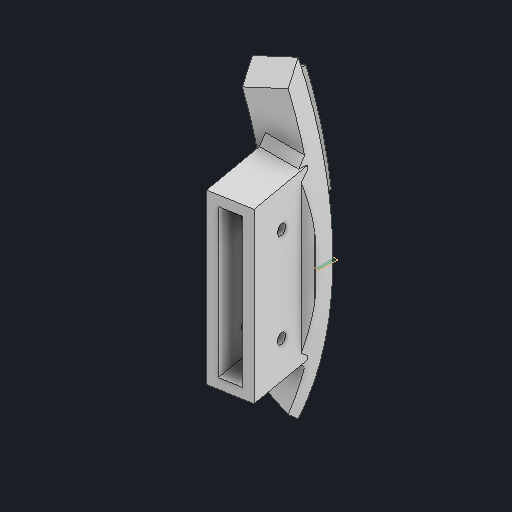
# Autodesk Inventor part: Lazercut_base
Saved by Autodesk Inventor 2023.4 (Build 274418000, 418)
## iProperties
Created: 2025-10-08
Part Number: Lazercut_base
Material: Generic
Document SubType Name: Modeling
Designer: Malthe Sennels
Density: 1 g/cm^3
Appearance: Default
Author: Malthe Sennels
Autodesk Inventor part; units mm, degrees
(part 1 of 2)
ref_plane "YZ Plane" through (0, 0, 0) normal (1, 0, 0) x (0, 1, 0)
ref_plane "XZ Plane" through (0, 0, 0) normal (0, 1, 0) x (-1, 0, 0)
ref_plane "XY Plane" through (0, 0, 0) normal (0, 0, 1) x (1, 0, 0)
sketch "Sketch1" plane through (0, 0, 0) normal (0, 0, 1) x (1, 0, 0)
  arc A0 (68.185975, 86.31728) -> (-68.185975, 86.31728) centre (0, 0) ccw
  arc A1 (5.434085, -92.914821) -> (6.399024, -89.470049) centre (-14.90414, -85.360206) ccw
  arc A2 (4.227461, -92.977534) -> (5.434085, -92.914821) centre (0, 0) ccw
  arc A3 (2.910609, -89.651355) -> (4.227461, -92.977534) centre (23.672934, -83.355206) ccw
  arc A4 (1.746562, -89.681585) -> (2.910609, -89.651355) centre (0, 0) ccw
  arc A5 (0.604127, -93.07163) -> (1.746562, -89.681585) centre (-19.314571, -84.471566) ccw
  arc A6 (-0.604127, -93.07163) -> (0.604127, -93.07163) centre (0, 0) ccw
  arc A7 (-1.746562, -89.681585) -> (-0.604127, -93.07163) centre (19.314571, -84.471566) ccw
  arc A8 (-2.910609, -89.651355) -> (-1.746562, -89.681585) centre (0, 0) ccw
  arc A9 (-4.227461, -92.977534) -> (-2.910609, -89.651355) centre (-23.672934, -83.355206) ccw
  arc A10 (-5.434085, -92.914821) -> (-4.227461, -92.977534) centre (0, 0) ccw
  arc A11 (-6.399024, -89.470049) -> (-5.434085, -92.914821) centre (14.90414, -85.360206) ccw
  arc A12 (-7.559934, -89.379442) -> (-6.399024, -89.470049) centre (0, 0) ccw
  arc A13 (-9.047651, -92.632787) -> (-7.559934, -89.379442) centre (-27.967478, -82.014135) ccw
  arc A14 (-10.249395, -92.50753) -> (-9.047651, -92.632787) centre (0, 0) ccw
  arc A15 (-11.034236, -89.017317) -> (-10.249395, -92.50753) centre (10.45353, -86.01873) ccw
  arc A16 (-12.188878, -88.866577) -> (-11.034236, -89.017317) centre (0, 0) ccw
  arc A17 (-13.843451, -92.038319) -> (-12.188878, -88.866577) centre (-32.186627, -80.451968) ccw
  arc A18 (-15.037073, -91.850856) -> (-13.843451, -92.038319) centre (0, 0) ccw
  arc A19 (-15.639701, -88.324611) -> (-15.037073, -91.850856) centre (5.974739, -86.445362) ccw
  arc A20 (-16.784963, -88.114143) -> (-15.639701, -88.324611) centre (0, 0) ccw
  arc A21 (-18.601932, -91.195731) -> (-16.784963, -88.114143) centre (-36.319007, -78.672917) ccw
  arc A22 (-19.784215, -90.946567) -> (-18.601932, -91.195731) centre (0, 0) ccw
  arc A23 (-20.203005, -87.393797) -> (-19.784215, -90.946567) centre (1.479841, -86.638954) ccw
  arc A24 (-21.335799, -87.124169) -> (-20.203005, -87.393797) centre (0, 0) ccw
  arc A25 (-23.310265, -90.107296) -> (-21.335799, -87.124169) centre (-40.353477, -76.681778) ccw
  arc A26 (-24.478021, -89.797103) -> (-23.310265, -90.107296) centre (0, 0) ccw
  arc A27 (-24.711845, -86.227385) -> (-24.478021, -89.797103) centre (-3.019046, -86.598981) ccw
  arc A28 (-25.829117, -85.899324) -> (-24.711845, -86.227385) centre (0, 0) ccw
  arc A29 (-27.955757, -88.775948) -> (-25.829117, -85.899324) centre (-44.279161, -74.483918) ccw
  arc A30 (-29.10584, -88.405562) -> (-27.955757, -88.775948) centre (0, 0) ccw
  arc A31 (-29.154066, -84.828519) -> (-29.10584, -88.405562) centre (-7.509794, -86.325554) ccw
  arc A32 (-30.252804, -84.44291) -> (-29.154066, -84.828519) centre (0, 0) ccw
  arc A33 (-32.525886, -87.205275) -> (-30.252804, -84.44291) centre (-48.085476, -72.085263) ccw
  arc A34 (-33.655194, -86.775695) -> (-32.525886, -87.205275) centre (0, 0) ccw
  arc A35 (-33.517693, -83.20097) -> (-33.655194, -86.775695) centre (-11.980297, -85.819407) ccw
  arc A36 (-34.594936, -82.758852) -> (-33.517693, -83.20097) centre (0, 0) ccw
  arc A37 (-37.008331, -85.399512) -> (-34.594936, -82.758852) centre (-51.762162, -69.492279) ccw
  arc A38 (-38.11382, -84.911896) -> (-37.008331, -85.399512) centre (0, 0) ccw
  arc A39 (-37.790962, -81.349126) -> (-38.11382, -84.911896) centre (-16.418504, -85.081907) ccw
  arc A40 (-38.843805, -80.851691) -> (-37.790962, -81.349126) centre (0, 0) ccw
  arc A41 (-41.391008, -83.363528) -> (-38.843805, -80.851691) centre (-55.299306, -66.711955) ccw
  arc A42 (-42.469697, -82.819189) -> (-41.391008, -83.363528) centre (0, 0) ccw
  arc A43 (-41.962354, -79.27798) -> (-42.469697, -82.819189) centre (-20.812449, -84.115041) ccw
  arc A44 (-42.987959, -78.726568) -> (-41.962354, -79.27798) centre (0, 0) ccw
  arc A45 (-45.662101, -81.10281) -> (-42.987959, -78.726568) centre (-58.687372, -63.751788) ccw
  arc A46 (-46.711084, -80.503217) -> (-45.662101, -81.10281) centre (0, 0) ccw
  arc A47 (-46.020622, -76.993114) -> (-46.711084, -80.503217) centre (-25.150288, -82.921416) ccw
  arc A48 (-47.016224, -76.389213) -> (-46.020622, -76.993114) centre (0, 0) ccw
  arc A49 (-49.810099, -78.623453) -> (-47.016224, -76.389213) centre (-61.917228, -60.619758) ccw
  arc A50 (-50.826546, -77.970222) -> (-49.810099, -78.623453) centre (0, 0) ccw
  arc A51 (-49.954827, -74.500688) -> (-50.826546, -77.970222) centre (-29.420325, -81.504249) ccw
  arc A52 (-50.917742, -73.845925) -> (-49.954827, -74.500688) centre (0, 0) ccw
  arc A53 (-53.823816, -75.932141) -> (-50.917742, -73.845925) centre (-64.980166, -57.324307) ccw
  arc A54 (-54.804988, -75.227033) -> (-53.823816, -75.932141) centre (0, 0) ccw
  arc A55 (-53.754362, -71.807421) -> (-54.804988, -75.227033) centre (-33.611051, -79.867362) ccw
  arc A56 (-54.681995, -71.103562) -> (-53.754362, -71.807421) centre (0, 0) ccw
  arc A57 (-57.692435, -73.03613) -> (-54.681995, -71.103562) centre (-67.867929, -53.874321) ccw
  arc A58 (-58.635686, -72.281046) -> (-57.692435, -73.03613) centre (0, 0) ccw
  arc A59 (-57.408985, -68.920574) -> (-58.635686, -72.281046) centre (-37.711167, -78.015166) ccw
  arc A60 (-58.298835, -68.169517) -> (-57.408985, -68.920574) centre (0, 0) ccw
  arc A61 (-61.405524, -69.943226) -> (-58.298835, -68.169517) centre (-70.572732, -50.279098) ccw
  arc A62 (-62.308313, -69.140201) -> (-61.405524, -69.943226) centre (0, 0) ccw
  arc A63 (-60.908844, -65.84793) -> (-62.308313, -69.140201) centre (-41.709621, -75.952654) ccw
  arc A64 (-61.758512, -65.051698) -> (-60.908844, -65.84793) centre (0, 0) ccw
  arc A65 (-64.953076, -66.661768) -> (-61.758512, -65.051698) centre (-73.087283, -46.548332) ccw
  arc A66 (-65.812967, -65.812967) -> (-64.953076, -66.661768) centre (0, 0) ccw
  arc A67 (-64.244503, -62.597771) -> (-65.812967, -65.812967) centre (-45.595633, -73.685388) ccw
  arc A68 (-65.051698, -61.758512) -> (-64.244503, -62.597771) centre (0, 0) ccw
  arc A69 (-68.325525, -63.200601) -> (-65.051698, -61.758512) centre (-75.404804, -42.69208) ccw
  arc A70 (-69.140201, -62.308313) -> (-68.325525, -63.200601) centre (0, 0) ccw
  arc A71 (-67.406971, -59.17886) -> (-69.140201, -62.308313) centre (-49.358727, -71.21948) ccw
  arc A72 (-68.169517, -58.298835) -> (-67.406971, -59.17886) centre (0, 0) ccw
  arc A73 (-71.513781, -59.569056) -> (-68.169517, -58.298835) centre (-77.519047, -38.720738) ccw
  arc A74 (-72.281046, -58.635686) -> (-71.513781, -59.569056) centre (0, 0) ccw
  arc A75 (-70.387721, -55.600413) -> (-72.281046, -58.635686) centre (-52.988759, -68.561576) ccw
  arc A76 (-71.103562, -54.681995) -> (-70.387721, -55.600413) centre (0, 0) ccw
  arc A77 (-74.509248, -55.776924) -> (-71.103562, -54.681995) centre (-79.424312, -34.645011) ccw
  arc A78 (-75.227033, -54.804988) -> (-74.509248, -55.776924) centre (0, 0) ccw
  arc A79 (-73.178718, -51.872077) -> (-75.227033, -54.804988) centre (-56.475942, -65.718842) ccw
  arc A80 (-73.845925, -50.917742) -> (-73.178718, -51.872077) centre (0, 0) ccw
  arc A81 (-77.303851, -51.834427) -> (-73.845925, -50.917742) centre (-81.115464, -30.475887) ccw
  arc A82 (-77.970222, -50.826546) -> (-77.303851, -51.834427) centre (0, 0) ccw
  arc A83 (-75.772439, -48.003903) -> (-77.970222, -50.826546) centre (-59.810876, -62.698942) ccw
  arc A84 (-76.389213, -47.016224) -> (-75.772439, -48.003903) centre (0, 0) ccw
  arc A85 (-79.890057, -47.752194) -> (-76.389213, -47.016224) centre (-82.587942, -26.224606) ccw
  arc A86 (-80.503217, -46.711084) -> (-79.890057, -47.752194) centre (0, 0) ccw
  arc A87 (-78.16189, -44.006319) -> (-80.503217, -46.711084) centre (-62.984571, -59.510016) ccw
  arc A88 (-78.726568, -42.987959) -> (-78.16189, -44.006319) centre (0, 0) ccw
  arc A89 (-82.260894, -43.541229) -> (-78.726568, -42.987959) centre (-83.837778, -21.902628) ccw
  arc A90 (-82.819189, -42.469697) -> (-82.260894, -43.541229) centre (0, 0) ccw
  arc A91 (-80.340631, -39.890102) -> (-82.819189, -42.469697) centre (-65.98847, -56.160662) ccw
  arc A92 (-80.851691, -38.843805) -> (-80.340631, -39.890102) centre (0, 0) ccw
  arc A93 (-84.409969, -39.212885) -> (-80.851691, -38.843805) centre (-84.861602, -17.521605) ccw
  arc A94 (-84.911896, -38.11382) -> (-84.409969, -39.212885) centre (0, 0) ccw
  arc A95 (-82.302787, -35.666348) -> (-84.911896, -38.11382) centre (-68.814477, -52.659909) ccw
  arc A96 (-82.758852, -34.594936) -> (-82.302787, -35.666348) centre (0, 0) ccw
  arc A97 (-86.331491, -34.77883) -> (-82.758852, -34.594936) centre (-85.656655, -13.093346) ccw
  arc A98 (-86.775695, -33.655194) -> (-86.331491, -34.77883) centre (0, 0) ccw
  arc A99 (-84.04307, -31.346444) -> (-86.775695, -33.655194) centre (-71.454971, -49.017194) ccw
  arc A100 (-84.44291, -30.252804) -> (-84.04307, -31.346444) centre (0, 0) ccw
  arc A101 (-88.020277, -30.251017) -> (-84.44291, -30.252804) centre (-86.220792, -8.62979) ccw
  arc A102 (-88.405562, -29.10584) -> (-88.020277, -30.251017) centre (0, 0) ccw
  arc A103 (-85.556787, -26.942036) -> (-88.405562, -29.10584) centre (-73.902836, -45.242337) ccw
  arc A104 (-85.899324, -25.829117) -> (-85.556787, -26.942036) centre (0, 0) ccw
  arc A105 (-89.471777, -25.641653) -> (-85.899324, -25.829117) centre (-86.552493, -4.142969) ccw
  arc A106 (-89.797103, -24.478021) -> (-89.471777, -25.641653) centre (0, 0) ccw
  arc A107 (-86.839859, -22.464997) -> (-89.797103, -24.478021) centre (-76.151471, -41.345515) ccw
  arc A108 (-87.124169, -21.335799) -> (-86.839859, -22.464997) centre (0, 0) ccw
  arc A109 (-90.682077, -20.963164) -> (-87.124169, -21.335799) centre (-86.650864, 0.35502) ccw
  arc A110 (-90.946567, -19.784215) -> (-90.682077, -20.963164) centre (0, 0) ccw
  arc A111 (-87.888826, -17.927395) -> (-90.946567, -19.784215) centre (-78.194816, -37.337233) ccw
  arc A112 (-88.114143, -16.784963) -> (-87.888826, -17.927395) centre (0, 0) ccw
  arc A113 (-91.647914, -16.228161) -> (-88.114143, -16.784963) centre (-86.515639, 4.852052) ccw
  arc A114 (-91.850856, -15.037073) -> (-91.647914, -16.228161) centre (0, 0) ccw
  arc A115 (-88.700859, -13.341465) -> (-91.850856, -15.037073) centre (-80.027361, -33.228296) ccw
  arc A116 (-88.866577, -12.188878) -> (-88.700859, -13.341465) centre (0, 0) ccw
  arc A117 (-92.366684, -11.44941) -> (-88.866577, -12.188878) centre (-86.147184, 9.336004) ccw
  arc A118 (-92.50753, -10.249395) -> (-92.366684, -11.44941) centre (0, 0) ccw
  arc A119 (-89.273772, -8.719569) -> (-92.50753, -10.249395) centre (-81.644167, -29.029782) ccw
  arc A120 (-89.379442, -7.559934) -> (-89.273772, -8.719569) centre (0, 0) ccw
  arc A121 (-92.83645, -6.639794) -> (-89.379442, -7.559934) centre (-85.546491, 13.794787) ccw
  arc A122 (-92.914821, -5.434085) -> (-92.83645, -6.639794) centre (0, 0) ccw
  arc A123 (-89.606017, -4.074166) -> (-92.914821, -5.434085) centre (-83.040874, -24.753008) ccw
  arc A124 (-89.651355, -2.910609) -> (-89.606017, -4.074166) centre (0, 0) ccw
  arc A125 (-93.055945, -1.812278) -> (-89.651355, -2.910609) centre (-84.715179, 18.216383) ccw
  arc A126 (-93.07163, -0.604127) -> (-93.055945, -1.812278) centre (0, 0) ccw
  arc A127 (-89.696701, 0.58222) -> (-93.07163, -0.604127) centre (-84.213718, -20.409505) ccw
  arc A128 (-89.681585, 1.746562) -> (-89.696701, 0.58222) centre (0, 0) ccw
  arc A129 (-93.024578, 3.020124) -> (-89.681585, 1.746562) centre (-83.655491, 22.58887) ccw
  arc A130 (-92.977534, 4.227461) -> (-93.024578, 3.020124) centre (0, 0) ccw
  arc A131 (-89.545578, 5.237036) -> (-92.977534, 4.227461) centre (-85.159537, -16.010981) ccw
  arc A132 (-89.470049, 6.399024) -> (-89.545578, 5.237036) centre (0, 0) ccw
  arc A133 (-92.742433, 7.844384) -> (-89.470049, 6.399024) centre (-82.370282, 26.900461) ccw
  arc A134 (-92.632787, 9.047651) -> (-92.742433, 7.844384) centre (0, 0) ccw
  arc A135 (-89.153057, 9.877735) -> (-92.632787, 9.047651) centre (-85.87578, -11.569295) ccw
  arc A136 (-89.017317, 11.034236) -> (-89.153057, 9.877735) centre (0, 0) ccw
  arc A137 (-92.210271, 12.647497) -> (-89.017317, 11.034236) centre (-80.863018, 31.139534) ccw
  arc A138 (-92.038319, 13.843451) -> (-92.210271, 12.647497) centre (0, 0) ccw
  arc A139 (-88.520194, 14.491805) -> (-92.038319, 13.843451) centre (-86.360518, -7.09642) ccw
  arc A140 (-88.324611, 15.639701) -> (-88.520194, 14.491805) centre (0, 0) ccw
  arc A141 (-91.429527, 17.416514) -> (-88.324611, 15.639701) centre (-79.137761, 35.29466) ccw
  arc A142 (-91.195731, 18.601932) -> (-91.429527, 17.416514) centre (0, 0) ccw
  arc A143 (-87.648697, 19.066807) -> (-91.195731, 18.601932) centre (-86.612443, -2.604414) ccw
  arc A144 (-87.393797, 20.203005) -> (-87.648697, 19.066807) centre (0, 0) ccw
  arc A145 (-90.402304, 22.13858) -> (-87.393797, 20.203005) centre (-77.199162, 39.354638) ccw
  arc A146 (-90.107296, 23.310265) -> (-90.402304, 22.13858) centre (0, 0) ccw
  arc A147 (-86.540914, 23.590409) -> (-90.107296, 23.310265) centre (-86.630876, 1.894613) ccw
  arc A148 (-86.227385, 24.711845) -> (-86.540914, 23.590409) centre (0, 0) ccw
  arc A149 (-89.131373, 26.800963) -> (-86.227385, 24.711845) centre (-75.052449, 43.308523) ccw
  arc A150 (-88.775948, 27.955757) -> (-89.131373, 26.800963) centre (0, 0) ccw
  arc A151 (-85.199832, 28.050415) -> (-88.775948, 27.955757) centre (-86.415767, 6.388533) ccw
  arc A152 (-84.828519, 29.154066) -> (-85.199832, 28.050415) centre (0, 0) ccw
  arc A153 (-87.620159, 31.391097) -> (-84.828519, 29.154066) centre (-72.703407, 47.145655) ccw
  arc A154 (-87.205275, 32.525886) -> (-87.620159, 31.391097) centre (0, 0) ccw
  arc A155 (-83.629067, 32.434802) -> (-87.205275, 32.525886) centre (-85.967697, 10.86523) ccw
  arc A156 (-83.20097, 33.517693) -> (-83.629067, 32.434802) centre (0, 0) ccw
  arc A157 (-85.872737, 35.896605) -> (-83.20097, 33.517693) centre (-70.15837, 50.855692) ccw
  arc A158 (-85.399512, 37.008331) -> (-85.872737, 35.896605) centre (0, 0) ccw
  arc A159 (-81.832852, 36.73175) -> (-85.399512, 37.008331) centre (-85.287874, 15.312636) ccw
  arc A160 (-81.349126, 37.790962) -> (-81.832852, 36.73175) centre (0, 0) ccw
  arc A161 (-83.893818, 40.305343) -> (-81.349126, 37.790962) centre (-67.424198, 54.42863) ccw
  arc A162 (-83.363528, 41.391008) -> (-83.893818, 40.305343) centre (0, 0) ccw
  arc A163 (-79.816031, 40.929677) -> (-83.363528, 41.391008) centre (-84.378129, 19.718762) ccw
  arc A164 (-79.27798, 41.962354) -> (-79.816031, 40.929677) centre (0, 0) ccw
  arc A165 (-81.688735, 44.605424) -> (-79.27798, 41.962354) centre (-64.508262, 57.854838) ccw
  arc A166 (-81.10281, 45.662101) -> (-81.688735, 44.605424) centre (0, 0) ccw
  arc A167 (-77.584039, 45.017264) -> (-81.10281, 45.662101) centre (-83.240915, 24.07173) ccw
  arc A168 (-76.993114, 46.020622) -> (-77.584039, 45.017264) centre (0, 0) ccw
  arc A169 (-79.263434, 48.785257) -> (-76.993114, 46.020622) centre (-61.418424, 61.12508) ccw
  arc A170 (-78.623453, 49.810099) -> (-79.263434, 48.785257) centre (0, 0) ccw
  arc A171 (-75.142895, 48.983492) -> (-78.623453, 49.810099) centre (-81.879299, 28.359805) ccw
  arc A172 (-74.500688, 49.954827) -> (-75.142895, 48.983492) centre (0, 0) ccw
  arc A173 (-76.624453, 52.833574) -> (-74.500688, 49.954827) centre (-58.163012, 64.23054) ccw
  arc A174 (-75.932141, 53.823816) -> (-76.624453, 52.833574) centre (0, 0) ccw
  arc A175 (-72.499179, 52.81767) -> (-75.932141, 53.823816) centre (-80.296951, 32.571427) ccw
  arc A176 (-71.807421, 53.754362) -> (-72.499179, 52.81767) centre (0, 0) ccw
  arc A177 (-73.778906, 56.73946) -> (-71.807421, 53.754362) centre (-54.750803, 67.162845) ccw
  arc A178 (-73.03613, 57.692435) -> (-73.778906, 56.73946) centre (0, 0) ccw
  arc A179 (-69.660017, 56.509461) -> (-73.03613, 57.692435) centre (-78.498136, 36.695242) ccw
  arc A180 (-68.920574, 57.408985) -> (-69.660017, 56.509461) centre (0, 0) ccw
  arc A181 (-70.734464, 60.492388) -> (-68.920574, 57.408985) centre (-51.190996, 69.914091) ccw
  arc A182 (-69.943226, 61.405524) -> (-70.734464, 60.492388) centre (0, 0) ccw
  arc A183 (-66.633065, 60.048912) -> (-69.943226, 61.405524) centre (-76.487705, 40.720133) ccw
  arc A184 (-65.84793, 60.908844) -> (-66.633065, 60.048912) centre (0, 0) ccw
  arc A185 (-67.499334, 64.082238) -> (-65.84793, 60.908844) centre (-47.493187, 72.476861) ccw
  arc A186 (-66.661768, 64.953076) -> (-67.499334, 64.082238) centre (0, 0) ccw
  arc A187 (-63.426482, 63.426482) -> (-66.661768, 64.953076) centre (-74.271076, 44.63525) ccw
  arc A188 (-62.597771, 64.244503) -> (-63.426482, 63.426482) centre (0, 0) ccw
  arc A189 (-64.082238, 67.499334) -> (-62.597771, 64.244503) centre (-43.667344, 74.844247) ccw
  arc A190 (-63.200601, 68.325525) -> (-64.082238, 67.499334) centre (0, 0) ccw
  arc A191 (-60.048912, 66.633065) -> (-63.200601, 68.325525) centre (-71.854225, 48.430038) ccw
  arc A192 (-59.17886, 67.406971) -> (-60.048912, 66.633065) centre (0, 0) ccw
  arc A193 (-60.492388, 70.734464) -> (-59.17886, 67.406971) centre (-39.723782, 77.009865) ccw
  arc A194 (-59.569056, 71.513781) -> (-60.492388, 70.734464) centre (0, 0) ccw
  arc A195 (-56.509461, 69.660017) -> (-59.569056, 71.513781) centre (-69.243668, 52.094267) ccw
  arc A196 (-55.600413, 70.387721) -> (-56.509461, 69.660017) centre (0, 0) ccw
  arc A197 (-56.73946, 73.778906) -> (-55.600413, 70.387721) centre (-35.673132, 78.967878) ccw
  arc A198 (-55.776924, 74.509248) -> (-56.73946, 73.778906) centre (0, 0) ccw
  arc A199 (-52.81767, 72.499179) -> (-55.776924, 74.509248) centre (-66.446442, 55.618059) ccw
  arc A200 (-51.872077, 73.178718) -> (-52.81767, 72.499179) centre (0, 0) ccw
  arc A201 (-52.833574, 76.624453) -> (-51.872077, 73.178718) centre (-31.526314, 80.713009) ccw
  arc A202 (-51.834427, 77.303851) -> (-52.833574, 76.624453) centre (0, 0) ccw
  arc A203 (-48.983492, 75.142895) -> (-51.834427, 77.303851) centre (-63.470089, 58.991915) ccw
  arc A204 (-48.003903, 75.772439) -> (-48.983492, 75.142895) centre (0, 0) ccw
  arc A205 (-48.785257, 79.263434) -> (-48.003903, 75.772439) centre (-27.294506, 82.240551) ccw
  arc A206 (-47.752194, 79.890057) -> (-48.785257, 79.263434) centre (0, 0) ccw
  arc A207 (-45.017264, 77.584039) -> (-47.752194, 79.890057) centre (-60.322631, 62.206739) ccw
  arc A208 (-44.006319, 78.16189) -> (-45.017264, 77.584039) centre (0, 0) ccw
  arc A209 (-44.605424, 81.688735) -> (-44.006319, 78.16189) centre (-22.989116, 83.546387) ccw
  arc A210 (-43.541229, 82.260894) -> (-44.605424, 81.688735) centre (0, 0) ccw
  arc A211 (-40.929677, 79.816031) -> (-43.541229, 82.260894) centre (-57.012554, 65.253865) ccw
  arc A212 (-39.890102, 80.340631) -> (-40.929677, 79.816031) centre (0, 0) ccw
  arc A213 (-40.305343, 83.893818) -> (-39.890102, 80.340631) centre (-18.621753, 84.626996) ccw
  arc A214 (-39.212885, 84.409969) -> (-40.305343, 83.893818) centre (0, 0) ccw
  arc A215 (-36.73175, 81.832852) -> (-39.212885, 84.409969) centre (-53.548782, 68.125078) ccw
  arc A216 (-35.666348, 82.302787) -> (-36.73175, 81.832852) centre (0, 0) ccw
  arc A217 (-35.896605, 85.872737) -> (-35.666348, 82.302787) centre (-14.204188, 85.479467) ccw
  arc A218 (-34.77883, 86.331491) -> (-35.896605, 85.872737) centre (0, 0) ccw
  arc A219 (-32.434802, 83.629067) -> (-34.77883, 86.331491) centre (-49.940651, 70.812637) ccw
  arc A220 (-31.346444, 84.04307) -> (-32.434802, 83.629067) centre (0, 0) ccw
  arc A221 (-31.391097, 87.620159) -> (-31.346444, 84.04307) centre (-9.748331, 86.1015) ccw
  arc A222 (-30.251017, 88.020277) -> (-31.391097, 87.620159) centre (0, 0) ccw
  arc A223 (-28.050415, 85.199832) -> (-30.251017, 88.020277) centre (-46.197889, 73.309298) ccw
  arc A224 (-26.942036, 85.556787) -> (-28.050415, 85.199832) centre (0, 0) ccw
  arc A225 (-26.800963, 89.131373) -> (-26.942036, 85.556787) centre (-5.266195, 86.491418) ccw
  arc A226 (-25.641653, 89.471777) -> (-26.800963, 89.131373) centre (0, 0) ccw
  arc A227 (-23.590409, 86.540914) -> (-25.641653, 89.471777) centre (-42.330586, 75.608331) ccw
  arc A228 (-22.464997, 86.839859) -> (-23.590409, 86.540914) centre (0, 0) ccw
  arc A229 (-22.13858, 90.402304) -> (-22.464997, 86.839859) centre (-0.769862, 86.648171) ccw
  arc A230 (-20.963164, 90.682077) -> (-22.13858, 90.402304) centre (0, 0) ccw
  arc A231 (-19.066807, 87.648697) -> (-20.963164, 90.682077) centre (-38.349167, 77.703537) ccw
  arc A232 (-17.927395, 87.888826) -> (-19.066807, 87.648697) centre (0, 0) ccw
  arc A233 (-17.416514, 91.429527) -> (-17.927395, 87.888826) centre (3.728547, 86.571336) ccw
  arc A234 (-16.228161, 91.647914) -> (-17.416514, 91.429527) centre (0, 0) ccw
  arc A235 (-14.491805, 88.520194) -> (-16.228161, 91.647914) centre (-34.264365, 79.589267) ccw
  arc A236 (-13.341465, 88.700859) -> (-14.491805, 88.520194) centre (0, 0) ccw
  arc A237 (-12.647497, 92.210271) -> (-13.341465, 88.700859) centre (8.216904, 86.261119) ccw
  arc A238 (-11.44941, 92.366684) -> (-12.647497, 92.210271) centre (0, 0) ccw
  arc A239 (-9.877735, 89.153057) -> (-11.44941, 92.366684) centre (-30.087193, 81.260439) ccw
  arc A240 (-8.719569, 89.273772) -> (-9.877735, 89.153057) centre (0, 0) ccw
  arc A241 (-7.844384, 92.742433) -> (-8.719569, 89.273772) centre (12.68311, 85.718358) ccw
  arc A242 (-6.639794, 92.83645) -> (-7.844384, 92.742433) centre (0, 0) ccw
  arc A243 (-5.237036, 89.545578) -> (-6.639794, 92.83645) centre (-25.828911, 82.712548) ccw
  arc A244 (-4.074166, 89.606017) -> (-5.237036, 89.545578) centre (0, 0) ccw
  arc A245 (-3.020124, 93.024578) -> (-4.074166, 89.606017) centre (17.115124, 84.944516) ccw
  arc A246 (-1.812278, 93.055945) -> (-3.020124, 93.024578) centre (0, 0) ccw
  arc A247 (-0.58222, 89.696701) -> (-1.812278, 93.055945) centre (-21.500999, 83.941678) ccw
  arc A248 (0.58222, 89.696701) -> (-0.58222, 89.696701) centre (0, 0) ccw
  arc A249 (1.812278, 93.055945) -> (0.58222, 89.696701) centre (21.500999, 83.941678) ccw
  arc A250 (3.020124, 93.024578) -> (1.812278, 93.055945) centre (0, 0) ccw
  arc A251 (4.074166, 89.606017) -> (3.020124, 93.024578) centre (-17.115124, 84.944516) ccw
  arc A252 (5.237036, 89.545578) -> (4.074166, 89.606017) centre (0, 0) ccw
  arc A253 (6.639794, 92.83645) -> (5.237036, 89.545578) centre (25.828911, 82.712548) ccw
  arc A254 (7.844384, 92.742433) -> (6.639794, 92.83645) centre (0, 0) ccw
  arc A255 (8.719569, 89.273772) -> (7.844384, 92.742433) centre (-12.68311, 85.718358) ccw
  arc A256 (9.877735, 89.153057) -> (8.719569, 89.273772) centre (0, 0) ccw
  arc A257 (11.44941, 92.366684) -> (9.877735, 89.153057) centre (30.087193, 81.260439) ccw
  arc A258 (12.647497, 92.210271) -> (11.44941, 92.366684) centre (0, 0) ccw
  arc A259 (13.341465, 88.700859) -> (12.647497, 92.210271) centre (-8.216904, 86.261119) ccw
  arc A260 (14.491805, 88.520194) -> (13.341465, 88.700859) centre (0, 0) ccw
  arc A261 (16.228161, 91.647914) -> (14.491805, 88.520194) centre (34.264365, 79.589267) ccw
  arc A262 (17.416514, 91.429527) -> (16.228161, 91.647914) centre (0, 0) ccw
  arc A263 (17.927395, 87.888826) -> (17.416514, 91.429527) centre (-3.728547, 86.571336) ccw
  arc A264 (19.066807, 87.648697) -> (17.927395, 87.888826) centre (0, 0) ccw
  arc A265 (20.963164, 90.682077) -> (19.066807, 87.648697) centre (38.349167, 77.703537) ccw
  arc A266 (22.13858, 90.402304) -> (20.963164, 90.682077) centre (0, 0) ccw
  arc A267 (22.464997, 86.839859) -> (22.13858, 90.402304) centre (0.769862, 86.648171) ccw
  arc A268 (23.590409, 86.540914) -> (22.464997, 86.839859) centre (0, 0) ccw
  arc A269 (25.641653, 89.471777) -> (23.590409, 86.540914) centre (42.330586, 75.608331) ccw
  arc A270 (26.800963, 89.131373) -> (25.641653, 89.471777) centre (0, 0) ccw
  arc A271 (26.942036, 85.556787) -> (26.800963, 89.131373) centre (5.266195, 86.491418) ccw
  arc A272 (28.050415, 85.199832) -> (26.942036, 85.556787) centre (0, 0) ccw
  arc A273 (30.251017, 88.020277) -> (28.050415, 85.199832) centre (46.197889, 73.309298) ccw
  arc A274 (31.391097, 87.620159) -> (30.251017, 88.020277) centre (0, 0) ccw
  arc A275 (31.346444, 84.04307) -> (31.391097, 87.620159) centre (9.748331, 86.1015) ccw
  arc A276 (32.434802, 83.629067) -> (31.346444, 84.04307) centre (0, 0) ccw
  arc A277 (34.77883, 86.331491) -> (32.434802, 83.629067) centre (49.940651, 70.812637) ccw
  arc A278 (35.896605, 85.872737) -> (34.77883, 86.331491) centre (0, 0) ccw
  arc A279 (35.666348, 82.302787) -> (35.896605, 85.872737) centre (14.204188, 85.479467) ccw
  arc A280 (36.73175, 81.832852) -> (35.666348, 82.302787) centre (0, 0) ccw
  arc A281 (39.212885, 84.409969) -> (36.73175, 81.832852) centre (53.548782, 68.125078) ccw
  arc A282 (40.305343, 83.893818) -> (39.212885, 84.409969) centre (0, 0) ccw
  arc A283 (39.890102, 80.340631) -> (40.305343, 83.893818) centre (18.621753, 84.626996) ccw
  arc A284 (40.929677, 79.816031) -> (39.890102, 80.340631) centre (0, 0) ccw
  arc A285 (43.541229, 82.260894) -> (40.929677, 79.816031) centre (57.012554, 65.253865) ccw
  arc A286 (44.605424, 81.688735) -> (43.541229, 82.260894) centre (0, 0) ccw
  arc A287 (44.006319, 78.16189) -> (44.605424, 81.688735) centre (22.989116, 83.546387) ccw
  arc A288 (45.017264, 77.584039) -> (44.006319, 78.16189) centre (0, 0) ccw
  arc A289 (47.752194, 79.890057) -> (45.017264, 77.584039) centre (60.322631, 62.206739) ccw
  arc A290 (48.785257, 79.263434) -> (47.752194, 79.890057) centre (0, 0) ccw
  arc A291 (48.003903, 75.772439) -> (48.785257, 79.263434) centre (27.294506, 82.240551) ccw
  arc A292 (48.983492, 75.142895) -> (48.003903, 75.772439) centre (0, 0) ccw
  arc A293 (51.834427, 77.303851) -> (48.983492, 75.142895) centre (63.470089, 58.991915) ccw
  arc A294 (52.833574, 76.624453) -> (51.834427, 77.303851) centre (0, 0) ccw
  arc A295 (51.872077, 73.178718) -> (52.833574, 76.624453) centre (31.526314, 80.713009) ccw
  arc A296 (52.81767, 72.499179) -> (51.872077, 73.178718) centre (0, 0) ccw
  arc A297 (55.776924, 74.509248) -> (52.81767, 72.499179) centre (66.446442, 55.618059) ccw
  arc A298 (56.73946, 73.778906) -> (55.776924, 74.509248) centre (0, 0) ccw
  arc A299 (55.600413, 70.387721) -> (56.73946, 73.778906) centre (35.673132, 78.967878) ccw
  arc A300 (56.509461, 69.660017) -> (55.600413, 70.387721) centre (0, 0) ccw
  arc A301 (59.569056, 71.513781) -> (56.509461, 69.660017) centre (69.243668, 52.094267) ccw
  arc A302 (60.492388, 70.734464) -> (59.569056, 71.513781) centre (0, 0) ccw
  arc A303 (59.17886, 67.406971) -> (60.492388, 70.734464) centre (39.723782, 77.009865) ccw
  arc A304 (60.048912, 66.633065) -> (59.17886, 67.406971) centre (0, 0) ccw
  arc A305 (63.200601, 68.325525) -> (60.048912, 66.633065) centre (71.854225, 48.430038) ccw
  arc A306 (64.082238, 67.499334) -> (63.200601, 68.325525) centre (0, 0) ccw
  arc A307 (62.597771, 64.244503) -> (64.082238, 67.499334) centre (43.667344, 74.844247) ccw
  arc A308 (63.426482, 63.426482) -> (62.597771, 64.244503) centre (0, 0) ccw
  arc A309 (66.661768, 64.953076) -> (63.426482, 63.426482) centre (74.271076, 44.63525) ccw
  arc A310 (67.499334, 64.082238) -> (66.661768, 64.953076) centre (0, 0) ccw
  arc A311 (65.84793, 60.908844) -> (67.499334, 64.082238) centre (47.493187, 72.476861) ccw
  arc A312 (66.633065, 60.048912) -> (65.84793, 60.908844) centre (0, 0) ccw
  arc A313 (69.943226, 61.405524) -> (66.633065, 60.048912) centre (76.487705, 40.720133) ccw
  arc A314 (70.734464, 60.492388) -> (69.943226, 61.405524) centre (0, 0) ccw
  arc A315 (68.920574, 57.408985) -> (70.734464, 60.492388) centre (51.190996, 69.914091) ccw
  arc A316 (69.660017, 56.509461) -> (68.920574, 57.408985) centre (0, 0) ccw
  arc A317 (73.03613, 57.692435) -> (69.660017, 56.509461) centre (78.498136, 36.695242) ccw
  arc A318 (73.778906, 56.73946) -> (73.03613, 57.692435) centre (0, 0) ccw
  arc A319 (71.807421, 53.754362) -> (73.778906, 56.73946) centre (54.750803, 67.162845) ccw
  arc A320 (72.499179, 52.81767) -> (71.807421, 53.754362) centre (0, 0) ccw
  arc A321 (75.932141, 53.823816) -> (72.499179, 52.81767) centre (80.296951, 32.571427) ccw
  arc A322 (76.624453, 52.833574) -> (75.932141, 53.823816) centre (0, 0) ccw
  arc A323 (74.500688, 49.954827) -> (76.624453, 52.833574) centre (58.163012, 64.23054) ccw
  arc A324 (75.142895, 48.983492) -> (74.500688, 49.954827) centre (0, 0) ccw
  arc A325 (78.623453, 49.810099) -> (75.142895, 48.983492) centre (81.879299, 28.359805) ccw
  arc A326 (79.263434, 48.785257) -> (78.623453, 49.810099) centre (0, 0) ccw
  arc A327 (76.993114, 46.020622) -> (79.263434, 48.785257) centre (61.418424, 61.12508) ccw
  arc A328 (77.584039, 45.017264) -> (76.993114, 46.020622) centre (0, 0) ccw
  arc A329 (81.10281, 45.662101) -> (77.584039, 45.017264) centre (83.240915, 24.07173) ccw
  arc A330 (81.688735, 44.605424) -> (81.10281, 45.662101) centre (0, 0) ccw
  arc A331 (79.27798, 41.962354) -> (81.688735, 44.605424) centre (64.508262, 57.854838) ccw
  arc A332 (79.816031, 40.929677) -> (79.27798, 41.962354) centre (0, 0) ccw
  arc A333 (83.363528, 41.391008) -> (79.816031, 40.929677) centre (84.378129, 19.718762) ccw
  arc A334 (83.893818, 40.305343) -> (83.363528, 41.391008) centre (0, 0) ccw
  arc A335 (81.349126, 37.790962) -> (83.893818, 40.305343) centre (67.424198, 54.42863) ccw
  arc A336 (81.832852, 36.73175) -> (81.349126, 37.790962) centre (0, 0) ccw
  arc A337 (85.399512, 37.008331) -> (81.832852, 36.73175) centre (85.287874, 15.312636) ccw
  arc A338 (85.872737, 35.896605) -> (85.399512, 37.008331) centre (0, 0) ccw
  arc A339 (83.20097, 33.517693) -> (85.872737, 35.896605) centre (70.15837, 50.855692) ccw
  arc A340 (83.629067, 32.434802) -> (83.20097, 33.517693) centre (0, 0) ccw
  arc A341 (87.205275, 32.525886) -> (83.629067, 32.434802) centre (85.967697, 10.86523) ccw
  arc A342 (87.620159, 31.391097) -> (87.205275, 32.525886) centre (0, 0) ccw
  arc A343 (84.828519, 29.154066) -> (87.620159, 31.391097) centre (72.703407, 47.145655) ccw
  arc A344 (85.199832, 28.050415) -> (84.828519, 29.154066) centre (0, 0) ccw
  arc A345 (88.775948, 27.955757) -> (85.199832, 28.050415) centre (86.415767, 6.388533) ccw
  arc A346 (89.131373, 26.800963) -> (88.775948, 27.955757) centre (0, 0) ccw
  arc A347 (86.227385, 24.711845) -> (89.131373, 26.800963) centre (75.052449, 43.308523) ccw
  arc A348 (86.540914, 23.590409) -> (86.227385, 24.711845) centre (0, 0) ccw
  arc A349 (90.107296, 23.310265) -> (86.540914, 23.590409) centre (86.630876, 1.894613) ccw
  arc A350 (90.402304, 22.13858) -> (90.107296, 23.310265) centre (0, 0) ccw
  arc A351 (87.393797, 20.203005) -> (90.402304, 22.13858) centre (77.199162, 39.354638) ccw
  arc A352 (87.648697, 19.066807) -> (87.393797, 20.203005) centre (0, 0) ccw
  arc A353 (91.195731, 18.601932) -> (87.648697, 19.066807) centre (86.612443, -2.604414) ccw
  arc A354 (91.429527, 17.416514) -> (91.195731, 18.601932) centre (0, 0) ccw
  arc A355 (88.324611, 15.639701) -> (91.429527, 17.416514) centre (79.137761, 35.29466) ccw
  arc A356 (88.520194, 14.491805) -> (88.324611, 15.639701) centre (0, 0) ccw
  arc A357 (92.038319, 13.843451) -> (88.520194, 14.491805) centre (86.360518, -7.09642) ccw
  arc A358 (92.210271, 12.647497) -> (92.038319, 13.843451) centre (0, 0) ccw
  arc A359 (89.017317, 11.034236) -> (92.210271, 12.647497) centre (80.863018, 31.139534) ccw
  arc A360 (89.153057, 9.877735) -> (89.017317, 11.034236) centre (0, 0) ccw
  arc A361 (92.632787, 9.047651) -> (89.153057, 9.877735) centre (85.87578, -11.569295) ccw
  arc A362 (92.742433, 7.844384) -> (92.632787, 9.047651) centre (0, 0) ccw
  arc A363 (89.470049, 6.399024) -> (92.742433, 7.844384) centre (82.370282, 26.900461) ccw
  arc A364 (89.545578, 5.237036) -> (89.470049, 6.399024) centre (0, 0) ccw
  arc A365 (92.977534, 4.227461) -> (89.545578, 5.237036) centre (85.159537, -16.010981) ccw
  arc A366 (93.024578, 3.020124) -> (92.977534, 4.227461) centre (0, 0) ccw
  arc A367 (89.681585, 1.746562) -> (93.024578, 3.020124) centre (83.655491, 22.58887) ccw
  arc A368 (89.696701, 0.58222) -> (89.681585, 1.746562) centre (0, 0) ccw
  arc A369 (93.07163, -0.604127) -> (89.696701, 0.58222) centre (84.213718, -20.409505) ccw
  arc A370 (93.055945, -1.812278) -> (93.07163, -0.604127) centre (0, 0) ccw
  arc A371 (89.651355, -2.910609) -> (93.055945, -1.812278) centre (84.715179, 18.216383) ccw
  arc A372 (89.606017, -4.074166) -> (89.651355, -2.910609) centre (0, 0) ccw
  arc A373 (92.914821, -5.434085) -> (89.606017, -4.074166) centre (83.040874, -24.753008) ccw
  arc A374 (92.83645, -6.639794) -> (92.914821, -5.434085) centre (0, 0) ccw
  arc A375 (89.379442, -7.559934) -> (92.83645, -6.639794) centre (85.546491, 13.794787) ccw
  arc A376 (89.273772, -8.719569) -> (89.379442, -7.559934) centre (0, 0) ccw
  arc A377 (92.50753, -10.249395) -> (89.273772, -8.719569) centre (81.644167, -29.029782) ccw
  arc A378 (92.366684, -11.44941) -> (92.50753, -10.249395) centre (0, 0) ccw
  arc A379 (88.866577, -12.188878) -> (92.366684, -11.44941) centre (86.147184, 9.336004) ccw
  arc A380 (88.700859, -13.341465) -> (88.866577, -12.188878) centre (0, 0) ccw
  arc A381 (91.850856, -15.037073) -> (88.700859, -13.341465) centre (80.027361, -33.228296) ccw
  arc A382 (91.647914, -16.228161) -> (91.850856, -15.037073) centre (0, 0) ccw
  arc A383 (88.114143, -16.784963) -> (91.647914, -16.228161) centre (86.515639, 4.852052) ccw
  arc A384 (87.888826, -17.927395) -> (88.114143, -16.784963) centre (0, 0) ccw
  arc A385 (90.946567, -19.784215) -> (87.888826, -17.927395) centre (78.194816, -37.337233) ccw
  arc A386 (90.682077, -20.963164) -> (90.946567, -19.784215) centre (0, 0) ccw
  arc A387 (87.124169, -21.335799) -> (90.682077, -20.963164) centre (86.650864, 0.35502) ccw
  arc A388 (86.839859, -22.464997) -> (87.124169, -21.335799) centre (0, 0) ccw
  arc A389 (89.797103, -24.478021) -> (86.839859, -22.464997) centre (76.151471, -41.345515) ccw
  arc A390 (89.471777, -25.641653) -> (89.797103, -24.478021) centre (0, 0) ccw
  arc A391 (85.899324, -25.829117) -> (89.471777, -25.641653) centre (86.552493, -4.142969) ccw
  arc A392 (85.556787, -26.942036) -> (85.899324, -25.829117) centre (0, 0) ccw
  arc A393 (88.405562, -29.10584) -> (85.556787, -26.942036) centre (73.902836, -45.242337) ccw
  arc A394 (88.020277, -30.251017) -> (88.405562, -29.10584) centre (0, 0) ccw
  arc A395 (84.44291, -30.252804) -> (88.020277, -30.251017) centre (86.220792, -8.62979) ccw
  arc A396 (84.04307, -31.346444) -> (84.44291, -30.252804) centre (0, 0) ccw
  arc A397 (86.775695, -33.655194) -> (84.04307, -31.346444) centre (71.454971, -49.017194) ccw
  arc A398 (86.331491, -34.77883) -> (86.775695, -33.655194) centre (0, 0) ccw
  arc A399 (82.758852, -34.594936) -> (86.331491, -34.77883) centre (85.656655, -13.093346) ccw
  arc A400 (82.302787, -35.666348) -> (82.758852, -34.594936) centre (0, 0) ccw
  arc A401 (84.911896, -38.11382) -> (82.302787, -35.666348) centre (68.814477, -52.659909) ccw
  arc A402 (84.409969, -39.212885) -> (84.911896, -38.11382) centre (0, 0) ccw
  arc A403 (80.851691, -38.843805) -> (84.409969, -39.212885) centre (84.861602, -17.521605) ccw
  arc A404 (80.340631, -39.890102) -> (80.851691, -38.843805) centre (0, 0) ccw
  arc A405 (82.819189, -42.469697) -> (80.340631, -39.890102) centre (65.98847, -56.160662) ccw
  arc A406 (82.260894, -43.541229) -> (82.819189, -42.469697) centre (0, 0) ccw
  arc A407 (78.726568, -42.987959) -> (82.260894, -43.541229) centre (83.837778, -21.902628) ccw
  arc A408 (78.16189, -44.006319) -> (78.726568, -42.987959) centre (0, 0) ccw
  arc A409 (80.503217, -46.711084) -> (78.16189, -44.006319) centre (62.984571, -59.510016) ccw
  arc A410 (79.890057, -47.752194) -> (80.503217, -46.711084) centre (0, 0) ccw
  arc A411 (76.389213, -47.016224) -> (79.890057, -47.752194) centre (82.587942, -26.224606) ccw
  arc A412 (75.772439, -48.003903) -> (76.389213, -47.016224) centre (0, 0) ccw
  arc A413 (77.970222, -50.826546) -> (75.772439, -48.003903) centre (59.810876, -62.698942) ccw
  arc A414 (77.303851, -51.834427) -> (77.970222, -50.826546) centre (0, 0) ccw
  arc A415 (73.845925, -50.917742) -> (77.303851, -51.834427) centre (81.115464, -30.475887) ccw
  arc A416 (73.178718, -51.872077) -> (73.845925, -50.917742) centre (0, 0) ccw
  arc A417 (75.227033, -54.804988) -> (73.178718, -51.872077) centre (56.475942, -65.718842) ccw
  arc A418 (74.509248, -55.776924) -> (75.227033, -54.804988) centre (0, 0) ccw
  arc A419 (71.103562, -54.681995) -> (74.509248, -55.776924) centre (79.424312, -34.645011) ccw
  arc A420 (70.387721, -55.600413) -> (71.103562, -54.681995) centre (0, 0) ccw
  arc A421 (72.281046, -58.635686) -> (70.387721, -55.600413) centre (52.988759, -68.561576) ccw
  arc A422 (71.513781, -59.569056) -> (72.281046, -58.635686) centre (0, 0) ccw
  arc A423 (68.169517, -58.298835) -> (71.513781, -59.569056) centre (77.519047, -38.720738) ccw
  arc A424 (67.406971, -59.17886) -> (68.169517, -58.298835) centre (0, 0) ccw
  arc A425 (69.140201, -62.308313) -> (67.406971, -59.17886) centre (49.358727, -71.21948) ccw
  arc A426 (68.325525, -63.200601) -> (69.140201, -62.308313) centre (0, 0) ccw
  arc A427 (65.051698, -61.758512) -> (68.325525, -63.200601) centre (75.404804, -42.69208) ccw
  arc A428 (64.244503, -62.597771) -> (65.051698, -61.758512) centre (0, 0) ccw
  arc A429 (65.812967, -65.812967) -> (64.244503, -62.597771) centre (45.595633, -73.685388) ccw
  arc A430 (64.953076, -66.661768) -> (65.812967, -65.812967) centre (0, 0) ccw
  arc A431 (61.758512, -65.051698) -> (64.953076, -66.661768) centre (73.087283, -46.548332) ccw
  arc A432 (60.908844, -65.84793) -> (61.758512, -65.051698) centre (0, 0) ccw
  arc A433 (62.308313, -69.140201) -> (60.908844, -65.84793) centre (41.709621, -75.952654) ccw
  arc A434 (61.405524, -69.943226) -> (62.308313, -69.140201) centre (0, 0) ccw
  arc A435 (58.298835, -68.169517) -> (61.405524, -69.943226) centre (70.572732, -50.279098) ccw
  arc A436 (57.408985, -68.920574) -> (58.298835, -68.169517) centre (0, 0) ccw
  arc A437 (58.635686, -72.281046) -> (57.408985, -68.920574) centre (37.711167, -78.015166) ccw
  arc A438 (57.692435, -73.03613) -> (58.635686, -72.281046) centre (0, 0) ccw
  arc A439 (54.681995, -71.103562) -> (57.692435, -73.03613) centre (67.867929, -53.874321) ccw
  arc A440 (53.754362, -71.807421) -> (54.681995, -71.103562) centre (0, 0) ccw
  arc A441 (54.804988, -75.227033) -> (53.754362, -71.807421) centre (33.611051, -79.867362) ccw
  arc A442 (53.823816, -75.932141) -> (54.804988, -75.227033) centre (0, 0) ccw
  arc A443 (50.917742, -73.845925) -> (53.823816, -75.932141) centre (64.980166, -57.324307) ccw
  arc A444 (49.954827, -74.500688) -> (50.917742, -73.845925) centre (0, 0) ccw
  arc A445 (50.826546, -77.970222) -> (49.954827, -74.500688) centre (29.420325, -81.504249) ccw
  arc A446 (49.810099, -78.623453) -> (50.826546, -77.970222) centre (0, 0) ccw
  arc A447 (47.016224, -76.389213) -> (49.810099, -78.623453) centre (61.917228, -60.619758) ccw
  arc A448 (46.020622, -76.993114) -> (47.016224, -76.389213) centre (0, 0) ccw
  arc A449 (46.711084, -80.503217) -> (46.020622, -76.993114) centre (25.150288, -82.921416) ccw
  arc A450 (45.662101, -81.10281) -> (46.711084, -80.503217) centre (0, 0) ccw
  arc A451 (42.987959, -78.726568) -> (45.662101, -81.10281) centre (58.687372, -63.751788) ccw
  arc A452 (41.962354, -79.27798) -> (42.987959, -78.726568) centre (0, 0) ccw
  arc A453 (42.469697, -82.819189) -> (41.962354, -79.27798) centre (20.812449, -84.115041) ccw
  arc A454 (41.391008, -83.363528) -> (42.469697, -82.819189) centre (0, 0) ccw
  arc A455 (38.843805, -80.851691) -> (41.391008, -83.363528) centre (55.299306, -66.711955) ccw
  arc A456 (37.790962, -81.349126) -> (38.843805, -80.851691) centre (0, 0) ccw
  arc A457 (38.11382, -84.911896) -> (37.790962, -81.349126) centre (16.418504, -85.081907) ccw
  arc A458 (37.008331, -85.399512) -> (38.11382, -84.911896) centre (0, 0) ccw
  arc A459 (34.594936, -82.758852) -> (37.008331, -85.399512) centre (51.762162, -69.492279) ccw
  arc A460 (33.517693, -83.20097) -> (34.594936, -82.758852) centre (0, 0) ccw
  arc A461 (33.655194, -86.775695) -> (33.517693, -83.20097) centre (11.980297, -85.819407) ccw
  arc A462 (32.525886, -87.205275) -> (33.655194, -86.775695) centre (0, 0) ccw
  arc A463 (30.252804, -84.44291) -> (32.525886, -87.205275) centre (48.085476, -72.085263) ccw
  arc A464 (29.154066, -84.828519) -> (30.252804, -84.44291) centre (0, 0) ccw
  arc A465 (29.10584, -88.405562) -> (29.154066, -84.828519) centre (7.509794, -86.325554) ccw
  arc A466 (27.955757, -88.775948) -> (29.10584, -88.405562) centre (0, 0) ccw
  arc A467 (25.829117, -85.899324) -> (27.955757, -88.775948) centre (44.279161, -74.483918) ccw
  arc A468 (24.711845, -86.227385) -> (25.829117, -85.899324) centre (0, 0) ccw
  arc A469 (24.478021, -89.797103) -> (24.711845, -86.227385) centre (3.019046, -86.598981) ccw
  arc A470 (23.310265, -90.107296) -> (24.478021, -89.797103) centre (0, 0) ccw
  arc A471 (21.335799, -87.124169) -> (23.310265, -90.107296) centre (40.353477, -76.681778) ccw
  arc A472 (20.203005, -87.393797) -> (21.335799, -87.124169) centre (0, 0) ccw
  arc A473 (19.784215, -90.946567) -> (20.203005, -87.393797) centre (-1.479841, -86.638954) ccw
  arc A474 (18.601932, -91.195731) -> (19.784215, -90.946567) centre (0, 0) ccw
  arc A475 (16.784963, -88.114143) -> (18.601932, -91.195731) centre (36.319007, -78.672917) ccw
  arc A476 (15.639701, -88.324611) -> (16.784963, -88.114143) centre (0, 0) ccw
  arc A477 (15.037073, -91.850856) -> (15.639701, -88.324611) centre (-5.974739, -86.445362) ccw
  arc A478 (13.843451, -92.038319) -> (15.037073, -91.850856) centre (0, 0) ccw
  arc A479 (12.188878, -88.866577) -> (13.843451, -92.038319) centre (32.186627, -80.451968) ccw
  arc A480 (11.034236, -89.017317) -> (12.188878, -88.866577) centre (0, 0) ccw
  arc A481 (10.249395, -92.50753) -> (11.034236, -89.017317) centre (-10.45353, -86.01873) ccw
  arc A482 (9.047651, -92.632787) -> (10.249395, -92.50753) centre (0, 0) ccw
  arc A483 (7.559934, -89.379442) -> (9.047651, -92.632787) centre (27.967478, -82.014135) ccw
  arc A484 (6.399024, -89.470049) -> (7.559934, -89.379442) centre (0, 0) ccw
  line L0 (-68.185975, 86.31728) -> (-81.31728, 86.31728)
  arc A485 (-81.31728, 86.31728) -> (-86.31728, 81.31728) centre (-81.31728, 81.31728) ccw
  line L1 (-86.31728, 81.31728) -> (-86.31728, 68.185975)
  arc A486 (-86.31728, 68.185975) -> (-86.31728, -68.185975) centre (0, 0) ccw
  line L2 (-86.31728, -68.185975) -> (-86.31728, -81.31728)
  arc A487 (-86.31728, -81.31728) -> (-81.31728, -86.31728) centre (-81.31728, -81.31728) ccw
  line L3 (-81.31728, -86.31728) -> (-68.185975, -86.31728)
  arc A488 (-68.185975, -86.31728) -> (68.185975, -86.31728) centre (0, 0) ccw
  line L4 (68.185975, -86.31728) -> (81.31728, -86.31728)
  arc A489 (81.31728, -86.31728) -> (86.31728, -81.31728) centre (81.31728, -81.31728) ccw
  line L5 (86.31728, -81.31728) -> (86.31728, -68.185975)
  arc A490 (86.31728, -68.185975) -> (86.31728, 68.185975) centre (0, 0) ccw
  line L6 (86.31728, 68.185975) -> (86.31728, 81.31728)
  arc A491 (86.31728, 81.31728) -> (81.31728, 86.31728) centre (81.31728, 81.31728) ccw
  line L7 (81.31728, 86.31728) -> (68.185975, 86.31728)
  arc A492 (68.185975, 86.31728) -> (-68.185975, 86.31728) centre (0, 0) ccw
  circle A493 centre (-81.31728, 81.31728) radius 3
  circle A494 centre (81.31728, 81.31728) radius 3
  circle A495 centre (-81.31728, -81.31728) radius 3
  circle A496 centre (81.31728, -81.31728) radius 3
  circle A497 centre (0, 0) radius 95
  line L8 (99.693857, 46.488009) -> (0, 0)
  line L9 (0, 0) -> (119.115415, 0)
  line L10 (99.693857, -46.488009) -> (0, 0)
  line L11 (-41.601173, -97.495346) -> (-39.24639, -91.976741)
  arc A498 (-39.24639, -91.976741) -> (-12.208077, -99.252017) centre (0, 0) ccw
  line L12 (-12.208077, -99.252017) -> (-12.940562, -105.207138)
  arc A499 (-41.601173, -97.495346) -> (-12.940562, -105.207138) centre (0, 0) ccw
  arc A500 (-12.208077, 99.252017) -> (-39.24639, 91.976741) centre (0, 0) ccw
  line L13 (-39.24639, 91.976741) -> (-41.601173, 97.495346)
  arc A501 (-12.940562, 105.207138) -> (-41.601173, 97.495346) centre (0, 0) ccw
  line L14 (-12.940562, 105.207138) -> (-12.208077, 99.252017)
  arc A502 (99.277389, 12) -> (92.058806, 39.053504) centre (0, 0) ccw
  line L15 (92.058806, 39.053504) -> (97.582335, 41.396714)
  arc A503 (105.234033, 12.72) -> (97.582335, 41.396714) centre (0, 0) ccw
  line L16 (105.234033, 12.72) -> (99.277389, 12)
  arc A504 (-79.85073, -60.198513) -> (-60.030999, -79.976741) centre (0, 0) ccw
  line L17 (-60.030999, -79.976741) -> (-63.632859, -84.775346)
  arc A505 (-84.641773, -63.810424) -> (-63.632859, -84.775346) centre (0, 0) ccw
  line L18 (-84.641773, -63.810424) -> (-79.85073, -60.198513)
  line L19 (-63.632859, 84.775346) -> (-60.030999, 79.976741)
  arc A506 (-60.030999, 79.976741) -> (-79.85073, 60.198513) centre (0, 0) ccw
  line L20 (-79.85073, 60.198513) -> (-84.641773, 63.810424)
  arc A507 (-63.632859, 84.775346) -> (-84.641773, 63.810424) centre (0, 0) ccw
  line L21 (97.582335, -41.396714) -> (92.058806, -39.053504)
  arc A508 (92.058806, -39.053504) -> (99.277389, -12) centre (0, 0) ccw
  line L22 (99.277389, -12) -> (105.234033, -12.72)
  arc A509 (97.582335, -41.396714) -> (105.234033, -12.72) centre (0, 0) ccw
  point P0 (86.09924, -40.148735)
  point P1 (86.09924, 40.148735)
  dimension "d0" = 15
  dimension "d1" = 25
  constraints: 6 end point, 1 centre point, 1 coincident, 1 horizontal, 1 point on circle, 1 symmetric about line
  measures "d0" radial gap between concentric circles of A490 A497
  measures "d1" angle of L9 L8
extrude "Extrusion1" add sketch "Sketch1" along normal blind 5 contours A490 L9 A497 L8 | A490 L10 A497 L9 | A502 L15 A503 L16 | L21 A508 L22 A509
ref_plane "Work Plane1" through (0, 0, 0) normal (0, -1, 0) x (1, 0, 0)
sketch "Sketch2" plane through (0, 0, 0) normal (0, -1, 0) x (1, 0, 0)
  line L0 (95, 5) -> (95, 0)
  line L1 (110, 0) -> (110, 5)
  line L2 (99.693857, 5) -> (99.693857, 5)
  line L3 (99.693857, 5) -> (86.09924, 5)
  line L4 (86.09924, 5) -> (86.09924, 5)
  line L5 (86.09924, 5) -> (99.693857, 5)
  line L6 (86.09924, 5) -> (95, 5)
  line L7 (110, 0) -> (95, 0)
  line L8 (95, 0) -> (95, 5)
  line L9 (95, 5) -> (110, 5)
  line L10 (110, 5) -> (110, 0)
  line L11 (98.236117, 6.076619) -> (101.70908, 25.772774)
  line L12 (101.70908, 25.772774) -> (107.814888, 24.696155)
  line L13 (107.814888, 24.696155) -> (104.341925, 5)
  line L14 (104.341925, 5) -> (98.236117, 6.076619)
  line L15 (106.775404, 1.524632) -> (111.290256, 27.129634)
  line L16 (111.290256, 27.129634) -> (99.275602, 29.248142)
  line L17 (99.275602, 29.248142) -> (94.760749, 3.64314)
  line L18 (94.760749, 3.64314) -> (106.775404, 1.524632)
  line L19 (107.814888, 24.696155) -> (110.769312, 24.175211)
  line L20 (101.70908, 25.772774) -> (98.754657, 26.293718)
  point P0 (0, 0)
  point P1 (107.388205, 5)
  dimension "d5" = 6.2
  dimension "d6" = 80
  dimension "d7" = 3
  dimension "d8" = 20
  constraints: 28 end point, 6 parallel, 6 point on line, 3 perpendicular, 1 horizontal, 3 other
  measures "d5" distance of L11.end L12.end
  measures "d6" angle of L9 L13
  measures "d7" distance between parallel lines of L13 L15
  measures "d8" distance of L12.end L13.end
extrude "Extrusion2" add sketch "Sketch2" along normal mid plane 50 contours L17 L20 L11 L14 L9 L3 | L13 L19 L15 L9
sketch "Sketch3" plane through (0, 25, 0) normal (0, 1, 0) x (1, 0, 0)
  line L0 (104.341925, -5) -> (107.814888, -24.696155)
  line L1 (107.814888, -24.696155) -> (110.769312, -24.175211)
  line L2 (110.769312, -24.175211) -> (107.388205, -5)
  line L3 (104.341925, -5) -> (107.121426, -5)
  line L4 (98.754657, -26.293718) -> (101.70908, -25.772774)
  line L5 (101.70908, -25.772774) -> (98.236117, -6.076619)
  line L6 (98.236117, -6.076619) -> (104.341925, -5)
  line L7 (95, -5) -> (104.341925, -5)
  line L8 (95, -5) -> (98.754657, -26.293718)
  line L9 (110.769312, -24.175211) -> (107.388205, -5)
  line L10 (95, -5) -> (98.754657, -26.293718)
  line L11 (110.769312, -24.175211) -> (98.754657, -26.293718)
  line L12 (98.754657, -26.293718) -> (95, -5)
  line L13 (95, -5) -> (107.014655, -2.881492)
  line L14 (107.014655, -2.881492) -> (110.769312, -24.175211)
  line L15 (107.388205, -5) -> (107.121426, -5)
  point P0 (0, 0)
  point P1 (106.169693, -5)
  point P2 (107.814888, -24.696155)
  constraints: 8 end point, 2 parallel, 2 perpendicular, 1 other
extrude "Extrusion3" add sketch "Sketch3" against normal blind 3 contours L0 L11 L5 L6
mirror "Mirror1" about plane through (0, 0, 0) normal (0, -1, 0) of "Extrusion3"
chamfer "Chamfer1" distance 5 angle 45 2 edges at (92.8965, 43.3184, 5) (92.8965, -43.3184, 5)
chamfer "Chamfer2" distance 2.25 angle 45 3 edges at (101.0607, 25, 5) (101.0607, -25, 5) (107.3882, 0, 5)